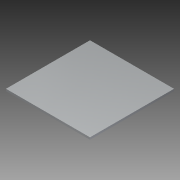
# Autodesk Inventor part: GLASS
Saved by Autodesk Inventor 2013 (Build 170138000, 138)
## iProperties
Created: 2014-03-03
Part Number: GLASS
Material: Generic
Document SubType Name: Modeling
Designer: employee
Density: 1 g/cm^3
Author: employee
Autodesk Inventor part; units mm, degrees
ref_plane "YZ Plane" through (0, 0, 0) normal (1, 0, 0) x (0, 1, 0)
ref_plane "XZ Plane" through (0, 0, 0) normal (0, 1, 0) x (-1, 0, 0)
ref_plane "XY Plane" through (0, 0, 0) normal (0, 0, 1) x (1, 0, 0)
sketch "Sketch1" plane through (0, 0, 0) normal (0, 0, 1) x (1, 0, 0)
  line L0 (-127, 127) -> (127, 127)
  line L1 (127, 127) -> (127, -127)
  line L2 (127, -127) -> (-127, -127)
  line L3 (-127, -127) -> (-127, 127)
  point P0 (0, 0)
  point P1 (0, 0)
  dimension "d0" = 254
  constraints: 8 end point, 1 coincident, 1 horizontal, 9 other
  measures "d0" distance of L0.start L0.end
extrude "Extrusion1" add sketch "Sketch1" along normal blind 6.35
body "Solid1"
